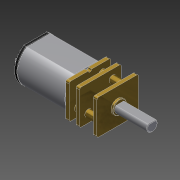
# Autodesk Inventor part: motor
Saved by Autodesk Inventor 2016 (Build 200138000, 138)
## iProperties
Created: 2011-07-06
Part Number: motor
Document SubType Name: Modeling
Designer: Patryk Antończyk
Density: 1 g/cm^3
Material: Generic
Appearance: Default
Author: Patryk Antończyk
Autodesk Inventor part; units mm, degrees
ref_plane "YZ Plane" through (0, 0, 0) normal (1, 0, 0) x (0, 1, 0)
ref_plane "XZ Plane" through (0, 0, 0) normal (0, 1, 0) x (-1, 0, 0)
ref_plane "XY Plane" through (0, 0, 0) normal (0, 0, 1) x (1, 0, 0)
sketch "Szkic1" plane through (0, 0, 0) normal (0, 0, 1) x (1, 0, 0)
  circle A0 centre (0, 0) radius 6
  line L0 (-3.3166, 5) -> (3.3166, 5)
  line L1 (-3.3166, -5) -> (3.3166, -5)
  line L2 (-6, 0) -> (6, 0)
  dimension "d0" = 12
  dimension "d1" = 10
  constraints: 6 end point, 6 point on circle, 2 parallel, 1 centre point, 1 coincident, 1 horizontal, 1 other
  measures "d0" diameter of A0
  measures "d1" distance between parallel lines of L0 L1
extrude "Wyciągnięcie proste1" add sketch "Szkic1" along normal blind 14 contours L2 A0 L0 | A0 L1 L2
fillet "Zaokrąglenie2" radius 0.25 4 edges at (0, 5, 14) (-6, 0, 14) (0, -5, 14) (6, 0, 14)
sketch "Szkic2" plane through (0, 0, 14) normal (0, 0, 1) x (1, 0, 0)
  line L0 (-6, 5) -> (6, 5)
  line L1 (6, 5) -> (6, -5)
  line L2 (6, -5) -> (-6, -5)
  line L3 (-6, -5) -> (-6, 5)
  constraints: 8 end point, 2 parallel, 1 horizontal, 1 perpendicular
extrude "Wyciągnięcie proste2" add sketch "Szkic2" along normal blind 1
fillet "Zaokrąglenie1" radius 0.5 4 edges at (-6, 5, 14.5) (-6, -5, 14.5) (6, -5, 14.5) (6, 5, 14.5)
sketch "Szkic3" plane through (0, 0, 15) normal (0, 0, 1) x (1, 0, 0)
  line L0 (-5.5, 5) -> (5.5, 5) projected
  circle A0 centre (0, 5) radius 0.5
  point P0 (0, 0)
  dimension "d7" = 1
  constraints: 1 centre point, 1 midpoint
  measures "d7" diameter of A0
extrude "Wyciągnięcie proste3" cut sketch "Szkic3" against normal blind 1
sketch "Szkic4" plane through (0, 0, 15) normal (0, 0, 1) x (1, 0, 0)
  line L0 (-6, -4.5) -> (-6, 4.5) projected
  line L1 (5.5, -5) -> (-5.5, -5) projected
  line L2 (6, 4.5) -> (6, -4.5) projected
  line L3 (0.5, 5) -> (5.5, 5) projected
  circle A0 centre (-3.5, -2.5) radius 1
  circle A1 centre (3.5, 2.5) radius 1
  point P0 (0, 0)
  dimension "d11" = 2
  dimension "d12" = 2
  dimension "d13" = 2.5
  dimension "d14" = 2.5
  dimension "d15" = 2.5
  dimension "d16" = 2.5
  constraints: 2 centre point
  measures "d11" diameter of A0
  measures "d12" diameter of A1
  measures "d13" distance from line of L2 A1.centre
  measures "d14" distance from line of L3 A1.centre
  measures "d15" distance from line of L0 A0.centre
  measures "d16" distance from line of L1 A0.centre
extrude "Wyciągnięcie proste4" add sketch "Szkic4" along normal blind 2
sketch "Szkic5" plane through (-3.5, -2.5, 17) normal (0, 0, 1) x (1, 0, 0)
  line L0 (-2.5, -2) -> (-2.5, 7) projected
  line L1 (-2, 7.5) -> (3, 7.5) projected
  line L2 (9, -2.5) -> (-2, -2.5) projected
  line L3 (9.5, 7) -> (9.5, -2) projected
  line L4 (-2.5, 7.5) -> (9.5, 7.5)
  line L5 (9.5, 7.5) -> (9.5, -2.5)
  line L6 (9.5, -2.5) -> (-2.5, -2.5)
  line L7 (-2.5, -2.5) -> (-2.5, 7.5)
  line L8 (9.5, -2.5) -> (4.5, -2.5)
  line L9 (4.5, -2.5) -> (4.5, 1.5)
  line L10 (4.5, 1.5) -> (9.5, 1.5)
  line L11 (9.5, 1.5) -> (9.5, -2.5)
  point P0 (3.5, 2.5)
  dimension "d19" = 5
  dimension "d20" = 4
  constraints: 16 end point, 4 parallel, 2 horizontal, 2 perpendicular
  measures "d19" distance of L9.end L10.end
  measures "d20" distance of L8.end L9.end
extrude "Wyciągnięcie proste5" add sketch "Szkic5" along normal blind 1 contours L0 L7 L4 L1 L5 L3 L10 L9 L2 L6
fillet "Zaokrąglenie3" radius 0.5 6 edges at (-6, -5, 17.5) (-6, 5, 17.5) (1, -5, 17.5) (1, -1, 17.5) (6, -1, 17.5) (6, 5, 17.5)
sketch "Szkic6" plane through (-3.5, -2.5, 18) normal (0, 0, 1) x (1, 0, 0)
  circle A0 centre (0, 0) radius 1 projected
  circle A1 centre (7, 5) radius 1 projected
  circle A2 centre (7, 5) radius 1 projected
  point P0 (3.5, 2.5)
extrude "Wyciągnięcie proste6" add sketch "Szkic6" along normal blind 4
sketch "Szkic7" plane through (-3.5, -2.5, 22) normal (0, 0, 1) x (1, 0, 0)
  line L0 (-2, 7.5) -> (9, 7.5) projected
  line L1 (-2.5, -2) -> (-2.5, 7) projected
  line L2 (4, -2.5) -> (-2, -2.5) projected
  line L3 (9.5, 7) -> (9.5, 2) projected
  line L4 (-2.5, 7.5) -> (9.5, 7.5)
  line L5 (9.5, 7.5) -> (9.5, -2.5)
  line L6 (9.5, -2.5) -> (-2.5, -2.5)
  line L7 (-2.5, -2.5) -> (-2.5, 7.5)
  point P0 (3.5, 2.5)
  constraints: 8 end point, 2 parallel, 1 horizontal, 1 perpendicular
extrude "Wyciągnięcie proste7" add sketch "Szkic7" along normal blind 1
fillet "Zaokrąglenie4" radius 0.5 4 edges at (-6, 5, 22.5) (-6, -5, 22.5) (6, -5, 22.5) (6, 5, 22.5)
sketch "Szkic8" plane through (-3.5, -2.5, 23) normal (0, 0, 1) x (1, 0, 0)
  circle A0 centre (3.5, 2.5) radius 1.95
  dimension "d29" = 3.9
  constraints: 1 centre point, 1 coincident
  measures "d29" diameter of A0
extrude "Wyciągnięcie proste8" add sketch "Szkic8" along normal blind 0.6
sketch "Szkic9" plane through (0, 0, 23.6) normal (0, 0, 1) x (1, 0, 0)
  circle A0 centre (0, 0) radius 1.95 projected
  circle A1 centre (0, 0) radius 1.5
  line L0 (-1.118, 1) -> (1.118, 1)
  dimension "d32" = 3
  dimension "d33" = 2.5
  constraints: 2 end point, 2 point on circle, 1 centre point, 1 coincident, 1 horizontal
  measures "d32" diameter of A1
extrude "Wyciągnięcie proste9" add sketch "Szkic9" along normal blind 9.4 contours A1 L0 picked at (0.0594, 0.1702)
chamfer "Faza1" distance 0.1 angle 45 1 edges at (-1.95, 0, 23.6)
chamfer "Faza2" distance 0.15 angle 45 2 edges at (0, 1, 33) (0, -1.5, 33)
fillet "Zaokrąglenie5" radius 0.1 4 edges at (0, 5, 0) (-6, 0, 0) (0, -5, 0) (6, 0, 0)
sketch "Szkic10" plane through (0, 0, 0) normal (0, 0, -1) x (-1, 0, 0)
  line L0 (3.3166, 5) -> (-3.3166, 5) projected
  arc A0 (-3.3166, 5) -> (-3.3166, -5) centre (0, 0) ccw projected
  arc A1 (3.3166, -5) -> (3.3166, 5) centre (0, 0) ccw projected
  line L1 (-3.3166, -5) -> (3.3166, -5) projected
extrude "Wyciągnięcie proste10" add sketch "Szkic10" along normal blind 1
fillet "Zaokrąglenie6" radius 0.1 4 edges at (0, 5, 0) (-6, 0, 0) (6, 0, 0) (0, -5, 0)
sketch "Szkic11" plane through (0, 0, -1) normal (0, 0, -1) x (-1, 0, 0)
  arc A0 (-3.3166, 5) -> (-3.3166, -5) centre (0, 0) ccw projected
  circle A1 centre (0, 0) radius 2.5
  dimension "d46" = 5
  constraints: 1 centre point, 1 coincident
  measures "d46" diameter of A1
extrude "Wyciągnięcie proste11" add sketch "Szkic11" along normal blind 0.5
hole "Hole1" at (0, 0, -1.5) direction (0, 0, 1) diameter 2 depth 0.2
sketch "Szkic13" plane through (0, 0, -1) normal (0, 0, -1) x (-1, 0, 0)
  circle A0 centre (0, 0) radius 2.5 projected
  line L0 (-3.6, 0.75) -> (-3.5, 0.75)
  line L1 (-3.5, 0.75) -> (-3.5, -0.75)
  line L2 (-3.5, -0.75) -> (-3.6, -0.75)
  line L3 (-3.6, -0.75) -> (-3.6, 0.75)
  point P0 (-3.5, 0)
  dimension "d58" = 0.1
  dimension "d59" = 1.5
  dimension "d60" = 3.5
  constraints: 8 end point, 2 parallel, 1 horizontal, 1 horizontal alignment, 1 midpoint, 1 perpendicular
  measures "d58" distance of L1.end L2.end
  measures "d59" distance of L0.end L1.end
  measures "d60" horizontal distance of A0.centre L1.end
extrude "Wyciągnięcie proste12" add sketch "Szkic13" along normal blind 2 contours L0 L1 L2 L3
fillet "Zaokrąglenie7" radius 0.25 2 edges at (3.55, 0.75, -3) (3.55, -0.75, -3)
sketch "Szkic14" plane through (3.5, -0.75, -1) normal (-1, 0, 0) x (0, 0, 1)
  line L0 (-2, 1.25) -> (-2, 0.25) projected
  line L1 (-1.4152, 0.85) -> (-1.1152, 0.85)
  line L2 (-1.0152, 0.75) -> (-1.0152, 0.75)
  line L3 (-1.1152, 0.65) -> (-1.4152, 0.65)
  line L4 (-1.5152, 0.75) -> (-1.5152, 0.75)
  arc A0 (-1.4152, 0.85) -> (-1.5152, 0.75) centre (-1.4152, 0.75) ccw
  arc A1 (-1.5152, 0.75) -> (-1.4152, 0.65) centre (-1.4152, 0.75) ccw
  arc A2 (-1.1152, 0.65) -> (-1.0152, 0.75) centre (-1.1152, 0.75) ccw
  arc A3 (-1.0152, 0.75) -> (-1.1152, 0.85) centre (-1.1152, 0.75) ccw
  point P0 (1, 0.75)
  point P1 (-1.0152, 0.65)
  point P2 (-1.0152, 0.85)
  point P3 (-1.5152, 0.65)
  point P4 (-1.5152, 0.75)
  point P5 (-2, 0.75)
  dimension "d64" = 0.5
  dimension "d65" = 0.2
  dimension "d66" = 0.1
  constraints: 8 end point, 8 point on circle, 8 tangent, 6 point on line, 4 centre point, 3 equal radius, 2 midpoint, 2 parallel, 1 horizontal, 1 horizontal alignment, 1 perpendicular
  measures "d64" distance of point (-1.015, 0.65) point (-1.515, 0.65)
  measures "d65" distance of point (-1.015, 0.85) point (-1.015, 0.65)
  measures "d66" radius of A0
extrude "Wyciągnięcie proste13" cut sketch "Szkic14" against normal through all
mirror "Odbicie lustrzane1" about plane through (0, 0, 0) normal (1, 0, 0) of "Wyciągnięcie proste12", "Zaokrąglenie7", "Wyciągnięcie proste13"
fillet "Zaokrąglenie8" radius 0.25 4 edges at (0, 5, -1) (6, 0, -1) (-6, 0, -1) (0, -5, -1)
fillet "Zaokrąglenie9" radius 0.1 2 edges at (2.5, 0, -1) (2.5, 0, -1.5)
fillet "Zaokrąglenie10" radius 0.1 1 edges at (0, -1, -1.5)
